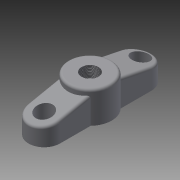
# Autodesk Inventor part: Base Superior
Saved by Autodesk Inventor 2015 (Build 190159000, 159)
## iProperties
Created: 2015-08-28
Part Number: Base Superior
Material: Generic
Document SubType Name: Modeling
Designer: EriveltonDell
Density: 1 g/cm^3
Appearance: Default
Author: EriveltonDell
Autodesk Inventor part; units mm, degrees
ref_plane "YZ Plane" through (0, 0, 0) normal (1, 0, 0) x (0, 1, 0)
ref_plane "XZ Plane" through (0, 0, 0) normal (0, 1, 0) x (-1, 0, 0)
ref_plane "XY Plane" through (0, 0, 0) normal (0, 0, 1) x (1, 0, 0)
sketch "Sketch5" plane through (0, 0, 0) normal (1, 0, 0) x (0, 1, 0)
  line L0 (0, 0) -> (0, 510)
  line L1 (0, 510) -> (70, 510)
  line L2 (70, 510) -> (70, 0)
  line L3 (70, 0) -> (0, 0)
  line L4 (0, 255) -> (110, 255)
  line L5 (110, 255) -> (110, 315)
  line L6 (110, 315) -> (70, 510)
  line L7 (110, 255) -> (110, 195)
  line L8 (110, 195) -> (70, 0)
  line L9 (0, 345) -> (0, 255)
  dimension "d9" = 510
  dimension "d10" = 70
  dimension "d11" = 510
  dimension "d12" = 110
  dimension "d13" = 60
  dimension "d14" = 60
  constraints: 20 end point, 2 perpendicular, 2 vertical, 1 midpoint, 1 parallel, 1 point on line
  measures "d9" distance of L0.start L0.end
  measures "d10" distance of L0.end L1.end
  measures "d11" distance of L1.end L2.end
  measures "d12" distance of L4.start L4.end
  measures "d13" distance of L4.end L5.end
  measures "d14" distance of L4.end L7.end
extrude "Extrusion4" add sketch "Sketch5" along normal blind 130
fillet "Fillet1" radius 65 4 edges at (130, 35, 510) (0, 35, 510) (130, 35, 0) (0, 35, 0)
sketch "Sketch6" plane through (0, 0, 65) normal (0, -1, 0) x (1, 0, 0)
  line L0 (0, -65) -> (65, -65)
  line L1 (65, -65) -> (65, 0)
  line L2 (65, 0) -> (65, 380)
  circle A0 centre (65, 380) radius 35
  circle A1 centre (65, -18.8688) radius 35
  circle A2 centre (65, 190) radius 35
  dimension "d20" = 65
  dimension "d21" = 65
  dimension "d22" = 380
  dimension "d23" = 70
  dimension "d24" = 70
  dimension "d25" = 70
  constraints: 6 end point, 3 centre point, 2 point on line, 1 coincident, 1 horizontal, 1 midpoint, 1 perpendicular
  measures "d20" distance of L0.start L0.end
  measures "d21" distance of L0.end L1.end
  measures "d22" distance of L1.end L2.end
  measures "d23" diameter of A0
  measures "d24" diameter of A1
  measures "d25" diameter of A2
extrude "Extrusion5" cut sketch "Sketch6" against normal through all
sketch "Sketch7" plane through (0, 0, 65) normal (0, -1, 0) x (1, 0, 0)
  line L0 (0, -65) -> (0, 190)
  line L1 (0, 130) -> (0, 250) projected
  line L2 (0, 190) -> (65, 190)
  circle A0 centre (65, 190) radius 90
  dimension "d28" = 65
  dimension "d29" = 180
  constraints: 4 end point, 1 centre point, 1 coincident, 1 horizontal, 1 midpoint
  measures "d28" distance of L0.end L2.end
  measures "d29" diameter of A0
extrude "Extrusion6" add sketch "Sketch7" against normal blind 130
sketch "Sketch8" plane through (65, 130, 255) normal (0, 1, 0) x (1, 0, 0)
  circle A0 centre (0, 0) radius 35
  point P0 (-65, 255)
  dimension "d32" = 70
  constraints: 1 centre point
  measures "d32" diameter of A0
extrude "Extrusion7" cut sketch "Sketch8" against normal blind 130
thread "Thread1" size "TR70x4" class "7H" standard "ISO Metric Trapezoidal Threads" full length
fillet "Fillet2" radius 10 1 edges at (-25, 130, 255)
fillet "Fillet3" radius 10 10 edges at (65, 70, 510) (110.962, 73.9052, 490.962) (19.038, 73.9052, 490.962) (0, 96.4359, 381.1248) (130, 96.4359, 381.1248) (19.038, 73.9052, 19.038) (110.962, 73.9052, 19.038) (65, 70, 0) (0, 96.4359, 128.8752) (130, 96.4359, 128.8752)
body "Solid2"
